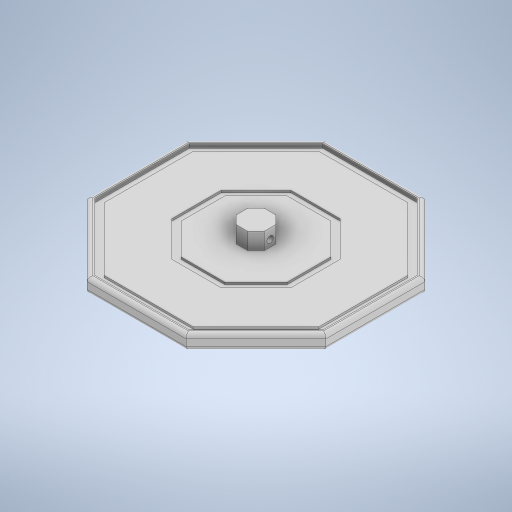
# Autodesk Inventor part: OV-PAM_bottom_2
Saved by Autodesk Inventor 2024 (Build 280153000, 153)
## iProperties
Created: 2023-06-16
Part Number: OV-PAM_bottom_2
Material: 일반
Document SubType Name: Modeling
Designer: jsw
Density: 1 g/cm^3
Appearance: 기본값
Author: jsw
Autodesk Inventor part; units mm, degrees
ref_plane "YZ Plane" through (0, 0, 0) normal (1, 0, 0) x (0, 1, 0)
ref_plane "XZ Plane" through (0, 0, 0) normal (0, 1, 0) x (-1, 0, 0)
ref_plane "XY Plane" through (0, 0, 0) normal (0, 0, 1) x (1, 0, 0)
sketch "스케치3" plane through (0, 0, 0) normal (0, 1, 0) x (-1, 0, 0)
  line L0 (35.7919, -14.8255) -> (14.8255, -35.7919)
  line L1 (14.8255, -35.7919) -> (-14.8255, -35.7919)
  line L2 (-14.8255, -35.7919) -> (-35.7919, -14.8255)
  line L3 (-35.7919, -14.8255) -> (-35.7919, 14.8255)
  line L4 (-35.7919, 14.8255) -> (-14.8255, 35.7919)
  line L5 (-14.8255, 35.7919) -> (14.8255, 35.7919)
  line L6 (14.8255, 35.7919) -> (35.7919, 14.8255)
  line L7 (35.7919, 14.8255) -> (35.7919, -14.8255)
  line L8 (13.5, -32.5919) -> (-13.5, -32.5919)
  line L9 (-13.5, -32.5919) -> (-32.5919, -13.5)
  line L10 (-32.5919, -13.5) -> (-32.5919, 13.5)
  line L11 (-32.5919, 13.5) -> (-13.5, 32.5919)
  line L12 (-13.5, 32.5919) -> (13.5, 32.5919)
  line L13 (13.5, 32.5919) -> (32.5919, 13.5)
  line L14 (32.5919, 13.5) -> (32.5919, -13.5)
  line L15 (32.5919, -13.5) -> (13.5, -32.5919)
  point P0 (0, 0)
  point P1 (0, 0)
  point P2 (0, 0)
  point P3 (0, 0)
  dimension "d66" = 27
  dimension "d67" = 3.2
  constraints: 32 end point, 3 coincident, 2 horizontal, 34 other
  measures "d66" distance of L8.start L8.end
  measures "d67" distance between parallel lines of L15 L0
extrude "돌출2" add sketch "스케치3" along normal blind 4.4 contours L0 L1 L2 L3 L4 L5 L6 L7 | L8 L9 L10 L11 L12 L13 L14 L15
sketch "스케치4" plane through (0, 4.4, 0) normal (0, 1, 0) x (1, 0, 0)
  line L0 (13.5, -32.5919) -> (-13.5, -32.5919)
  line L1 (-13.5, -32.5919) -> (-32.5919, -13.5)
  line L2 (-32.5919, -13.5) -> (-32.5919, 13.5)
  line L3 (-32.5919, 13.5) -> (-13.5, 32.5919)
  line L4 (-13.5, 32.5919) -> (13.5, 32.5919)
  line L5 (13.5, 32.5919) -> (32.5919, 13.5)
  line L6 (32.5919, 13.5) -> (32.5919, -13.5)
  line L7 (32.5919, -13.5) -> (13.5, -32.5919)
  line L8 (-14.1627, 34.1919) -> (14.1627, 34.1919)
  line L9 (14.1627, 34.1919) -> (34.1919, 14.1627)
  line L10 (34.1919, 14.1627) -> (34.1919, -14.1627)
  line L11 (34.1919, -14.1627) -> (14.1627, -34.1919)
  line L12 (14.1627, -34.1919) -> (-14.1627, -34.1919)
  line L13 (-14.1627, -34.1919) -> (-34.1919, -14.1627)
  line L14 (-34.1919, -14.1627) -> (-34.1919, 14.1627)
  line L15 (-34.1919, 14.1627) -> (-14.1627, 34.1919)
  line L16 (-13.3343, 32.1919) -> (13.3343, 32.1919)
  line L17 (13.3343, 32.1919) -> (32.1919, 13.3343)
  line L18 (32.1919, 13.3343) -> (32.1919, -13.3343)
  line L19 (32.1919, -13.3343) -> (13.3343, -32.1919)
  line L20 (13.3343, -32.1919) -> (-13.3343, -32.1919)
  line L21 (-13.3343, -32.1919) -> (-32.1919, -13.3343)
  line L22 (-32.1919, -13.3343) -> (-32.1919, 13.3343)
  line L23 (-32.1919, 13.3343) -> (-13.3343, 32.1919)
  line L24 (-14.8255, 35.7919) -> (-35.7919, 14.8255) projected
  point P0 (0, 0)
  point P1 (0, 0)
  point P2 (0, 0)
  point P3 (0, 0)
  dimension "d7" = 27
  dimension "d110" = 1.6
  dimension "d111" = 2
  constraints: 48 end point, 3 coincident, 3 horizontal, 51 other
  measures "d7" distance of L1.end L2.end
  measures "d110" distance between parallel lines of L15 L24
  measures "d111" distance between parallel lines of L15 L23
extrude "돌출3" cut sketch "스케치4" against normal blind 1.2 contours L0 L1 L2 L3 L4 L5 L6 L7 | L8 L9 L10 L11 L12 L13 L14 L15 | L16 L17 L18 L19 L20 L21 L22 L23
sketch "스케치9" plane through (0, 0, 0) normal (0, -1, 0) x (1, 0, 0)
  line L0 (7.5, 10) -> (2.5, 10)
  line L1 (2.5, 10) -> (2.5, -10)
  line L2 (2.5, -10) -> (7.5, -10)
  line L3 (7.5, -10) -> (7.5, 10)
  line L4 (7.5, 10) -> (2.5, -10) construction
  line L5 (2.5, 10) -> (7.5, -10) construction
  line L6 (-2.5, 10) -> (-7.5, 10)
  line L7 (-7.5, 10) -> (-7.5, -10)
  line L8 (-7.5, -10) -> (-2.5, -10)
  line L9 (-2.5, 10) -> (-7.5, -10) construction
  line L10 (-7.5, 10) -> (-2.5, -10) construction
  line L11 (-2.5, -10) -> (-2.5, 10)
  point P0 (0, 0)
  point P1 (5, 0)
  point P2 (-5, 0)
  dimension "d42" = 20
  dimension "d43" = 5
  dimension "d44" = 2.5
  dimension "d47" = 10
  constraints: 24 end point, 2 horizontal, 2 midpoint, 2 parallel, 1 collinear, 1 horizontal alignment, 1 perpendicular, 10 other
  measures "d42" distance of L2.end L0.start
  measures "d43" distance of L1.end L2.end
  measures "d44" distance from line of L1 point (0, 0)
  measures "d47" distance of L0.start L6.start
extrude "돌출8" add sketch "스케치9" along normal blind 10
sketch "스케치10" plane through (-7.5, 0, -10) normal (-1, 0, 0) x (0, 0, 1)
  circle A0 centre (15, -5) radius 1.25
  line L0 (19.9591, 0) -> (0.0886, 0)
  line L1 (24.8255, 0) -> (-4.8255, 0) projected
  circle A1 centre (5, -5) radius 1.25
  line L2 (20, 0) -> (20, -10) projected
  point P0 (10, 0)
  dimension "d54" = 2.5
  dimension "d57" = 10
  dimension "d62" = 5
  dimension "d63" = 5
  constraints: 2 centre point, 2 end point, 1 horizontal, 1 point on line, 2 other
  measures "d54" diameter of A0
  measures "d57" distance of A0.centre A1.centre
  measures "d62" distance from line of L0 A0.centre
  measures "d63" distance from line of L2 A0.centre
extrude "돌출9" cut sketch "스케치10" against normal blind 20
sketch "스케치11" plane through (0, 3.2, 0) normal (0, 1, 0) x (1, 0, 0)
  line L0 (-13.3343, 32.1919) -> (13.3343, 32.1919)
  line L1 (13.3343, 32.1919) -> (32.1919, 13.3343)
  line L2 (32.1919, 13.3343) -> (32.1919, -13.3343)
  line L3 (32.1919, -13.3343) -> (13.3343, -32.1919)
  line L4 (13.3343, -32.1919) -> (-13.3343, -32.1919)
  line L5 (-13.3343, -32.1919) -> (-32.1919, -13.3343)
  line L6 (-32.1919, -13.3343) -> (-32.1919, 13.3343)
  line L7 (-32.1919, 13.3343) -> (-13.3343, 32.1919)
  line L8 (-14.1627, 34.1919) -> (14.1627, 34.1919) projected
  line L9 (-12.0917, 29.1919) -> (12.0917, 29.1919)
  line L10 (12.0917, 29.1919) -> (29.1919, 12.0917)
  line L11 (29.1919, 12.0917) -> (29.1919, -12.0917)
  line L12 (29.1919, -12.0917) -> (12.0917, -29.1919)
  line L13 (12.0917, -29.1919) -> (-12.0917, -29.1919)
  line L14 (-12.0917, -29.1919) -> (-29.1919, -12.0917)
  line L15 (-29.1919, -12.0917) -> (-29.1919, 12.0917)
  line L16 (-29.1919, 12.0917) -> (-12.0917, 29.1919)
  point P0 (0, 0)
  point P1 (0, 0)
  point P2 (0, 0)
  dimension "d70" = 2
  dimension "d71" = 3
  constraints: 32 end point, 2 coincident, 2 horizontal, 34 other
  measures "d70" distance between parallel lines of L8 L0
  measures "d71" distance between parallel lines of L9 L0
extrude "돌출10" add sketch "스케치11" along normal blind 0.6 contours L0 L1 L2 L3 L4 L5 L6 L7 | L9 L10 L11 L12 L13 L14 L15 L16
fillet "모깎기1" radius 1.2 16 edges at (-25.3087, 4.4, 25.3087) (0, 4.4, 35.7919) (25.3087, 4.4, 25.3087) (35.7919, 4.4, 0) (25.3087, 4.4, -25.3087) (0, 4.4, -35.7919) (-25.3087, 4.4, -25.3087) (-35.7919, 4.4, 0) (-25.3087, 0, 25.3087) (0, 0, 35.7919) (25.3087, 0, 25.3087) (35.7919, 0, 0) (25.3087, 0, -25.3087) (0, 0, -35.7919) (-25.3087, 0, -25.3087) (-35.7919, 0, 0)
sketch "스케치13" plane through (0, 3.8, 0) normal (0, 1, 0) x (1, 0, 0)
  line L0 (-6.575, 15.8735) -> (6.575, 15.8735)
  line L1 (6.575, 15.8735) -> (15.8735, 6.575)
  line L2 (15.8735, 6.575) -> (15.8735, -6.575)
  line L3 (15.8735, -6.575) -> (6.575, -15.8735)
  line L4 (6.575, -15.8735) -> (-6.575, -15.8735)
  line L5 (-6.575, -15.8735) -> (-15.8735, -6.575)
  line L6 (-15.8735, -6.575) -> (-15.8735, 6.575)
  line L7 (-15.8735, 6.575) -> (-6.575, 15.8735)
  line L8 (-7.4034, 17.8735) -> (7.4034, 17.8735)
  line L9 (7.4034, 17.8735) -> (17.8735, 7.4034)
  line L10 (17.8735, 7.4034) -> (17.8735, -7.4034)
  line L11 (17.8735, -7.4034) -> (7.4034, -17.8735)
  line L12 (7.4034, -17.8735) -> (-7.4034, -17.8735)
  line L13 (-7.4034, -17.8735) -> (-17.8735, -7.4034)
  line L14 (-17.8735, -7.4034) -> (-17.8735, 7.4034)
  line L15 (-17.8735, 7.4034) -> (-7.4034, 17.8735)
  point P0 (0, 0)
  point P1 (0, 0)
  point P2 (0, 0)
  dimension "d99" = 13.15
  dimension "d100" = 2
  constraints: 32 end point, 2 coincident, 2 horizontal, 34 other
  measures "d99" distance of L0.start L0.end
  measures "d100" distance between parallel lines of L0 L8
extrude "돌출11" cut sketch "스케치13" against normal blind 0.6
sketch "스케치14" plane through (0, 3.8, 0) normal (0, 1, 0) x (1, 0, 0)
  line L0 (-1.75, 4.2249) -> (1.75, 4.2249)
  line L1 (1.75, 4.2249) -> (4.2249, 1.75)
  line L2 (4.2249, 1.75) -> (4.2249, -1.75)
  line L3 (4.2249, -1.75) -> (1.75, -4.2249)
  line L4 (1.75, -4.2249) -> (-1.75, -4.2249)
  line L5 (-1.75, -4.2249) -> (-4.2249, -1.75)
  line L6 (-4.2249, -1.75) -> (-4.2249, 1.75)
  line L7 (-4.2249, 1.75) -> (-1.75, 4.2249)
  point P0 (0, 0)
  point P1 (0, 0)
  dimension "d103" = 3.5
  constraints: 16 end point, 1 coincident, 1 horizontal, 17 other
  measures "d103" distance of L1.end L2.end
extrude "돌출12" add sketch "스케치14" along normal blind 5
sketch "스케치16" plane through (-4.2249, 3.8, -1.75) normal (-1, 0, 0) x (0, 0, 1)
  circle A0 centre (1.75, 2) radius 1
  line L0 (3.5, 0) -> (0, 0) projected
  point P0 (1.75, -3.8)
  dimension "d106" = 2
  dimension "d107" = 2
  constraints: 1 centre point
  measures "d106" diameter of A0
  measures "d107" distance from line of L0 A0.centre
extrude "돌출13" cut sketch "스케치16" against normal up to surface (8.4497 mm away)
